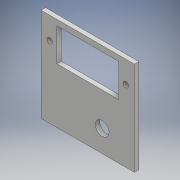
# Autodesk Inventor part: mocowanie ostatniego serwa
Saved by Autodesk Inventor 2017.3 (Build 213256000, 256)
## iProperties
Created: 2019-03-17
Part Number: mocowanie ostatniego serwa
Material: Ogólny
Document SubType Name: Modeling
Designer: legox
Density: 1 g/cm^3
Appearance: Domyślna
Author: legox
Autodesk Inventor part; units mm, degrees
ref_plane "YZ Plane" through (0, 0, 0) normal (1, 0, 0) x (0, 1, 0)
ref_plane "XZ Plane" through (0, 0, 0) normal (0, 1, 0) x (-1, 0, 0)
ref_plane "XY Plane" through (0, 0, 0) normal (0, 0, 1) x (1, 0, 0)
sketch "Szkic1" plane through (0, 0, 0) normal (0, 1, 0) x (-1, 0, 0)
  line L0 (0, 0) -> (-34, 0)
  line L1 (-34, 0) -> (-34, -34.1)
  line L2 (-34, -34.1) -> (0, -34.1)
  line L3 (0, -34.1) -> (0, 0)
  line L4 (-5.75, -2) -> (-28.25, -2)
  line L5 (-28.25, -2) -> (-28.25, -14)
  line L6 (-28.25, -14) -> (-5.75, -14)
  line L7 (-5.75, -14) -> (-5.75, -2)
  circle A0 centre (-3.15, -8) radius 1
  circle A1 centre (-30.85, -8) radius 1
  dimension "d0" = 34
  dimension "d1" = 34.1
  dimension "d2" = 22.5
  dimension "d3" = 12
  dimension "d4" = 2
  dimension "d5" = 5.75
  dimension "d6" = 2
  dimension "d7" = 2.6
  dimension "d8" = 2
  dimension "d9" = 2.6
  dimension "d12" = 6
  dimension "d13" = 6
  constraints: 16 end point, 4 parallel, 2 centre point, 2 horizontal, 2 perpendicular
  measures "d0" distance of L2.end L1.end
  measures "d1" distance of L0.end L1.end
  measures "d2" distance of L6.end L5.end
  measures "d3" distance of L5.end L4.end
  measures "d4" distance between parallel lines of L0 L4
  measures "d5" distance between parallel lines of L1 L5
  measures "d6" diameter of A0
  measures "d7" distance from line of L7 A0.centre
  measures "d8" diameter of A1
  measures "d9" distance from line of L5 A1.centre
  measures "d12" distance from line of L4 A1.centre
  measures "d13" distance from line of L4 A0.centre
extrude "Wyciągnięcie proste1" add sketch "Szkic1" along normal blind 1.6
sketch "Szkic2" plane through (0, 1.6, 0) normal (0, 1, 0) x (1, 0, 0)
  circle A0 centre (22.25, 26.1) radius 2.5
  line L0 (34, 0) -> (34, 34.1) projected
  line L1 (34, 34.1) -> (0, 34.1) projected
  point P0 (0, 0)
  dimension "d14" = 5
  dimension "d15" = 11.75
  dimension "d16" = 8
  constraints: 1 centre point
  measures "d14" diameter of A0
  measures "d15" distance from line of L0 A0.centre
  measures "d16" distance from line of L1 A0.centre
extrude "Wyciągnięcie proste2" cut sketch "Szkic2" against normal blind 1.6
equation "\"d5\" = -0.5 * d2 + 0.5 * d0"
equation "\"d12\" = 0.5 * d3"
equation "\"d13\" = d12"
